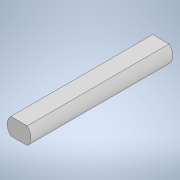
# Autodesk Inventor part: wheel_axle
Saved by Autodesk Inventor 2020.3 (Build 243373000, 373)
## iProperties
Created: 2020-06-20
Part Number: wheel_axle
Material: Generic
Document SubType Name: Modeling
Designer: Devin
Density: 1 g/cm^3
Appearance: Default
Author: Devin
Autodesk Inventor part; units mm, degrees
ref_plane "YZ Plane" through (0, 0, 0) normal (1, 0, 0) x (0, 1, 0)
ref_plane "XZ Plane" through (0, 0, 0) normal (0, 1, 0) x (-1, 0, 0)
ref_plane "XY Plane" through (0, 0, 0) normal (0, 0, 1) x (1, 0, 0)
sketch "Sketch1" plane through (0, 0, 0) normal (0, 0, 1) x (1, 0, 0)
  line L0 (-1.7349, -1.8) -> (1.7349, -1.8)
  line L1 (1.7349, 1.8) -> (-1.7349, 1.8)
  arc A0 (-1.7349, 1.8) -> (-1.7349, -1.8) centre (0, 0) ccw
  arc A1 (1.7349, -1.8) -> (1.7349, 1.8) centre (0, 0) ccw
  constraints: 4 end point, 4 point on circle, 2 centre point, 2 horizontal
extrude "Extrusion1" add sketch "Sketch1" along normal blind 30
body "Solid1"
